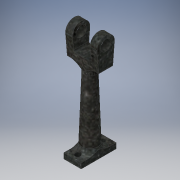
# Autodesk Inventor part: Crankrod
Saved by Autodesk Inventor 2017 (Build 210142000, 142)
## iProperties
Created: 2018-11-07
Part Number: Crankrod
Material: Steel
Document SubType Name: Modeling
Designer: 623516
Density: 7.85 g/cm^3
Appearance: Plate
Author: 623516
Autodesk Inventor part; units mm, degrees
ref_plane "YZ Plane" through (0, 0, 0) normal (1, 0, 0) x (0, 1, 0)
sketch "Sketch1" plane through (0, 0, 0) normal (0, 1, 0) x (-1, 0, 0)
  line L0 (0, 0) -> (10, 0)
  line L1 (10, 0) -> (10, 20)
  line L2 (10, 20) -> (0, 20)
  line L3 (0, 20) -> (0, 0)
  dimension "d0" = 10
  dimension "d1" = 20
  constraints: 8 end point, 2 parallel, 1 horizontal, 1 perpendicular
  measures "d0" distance of L2.end L1.end
  measures "d1" distance of L1.end L0.end
extrude "Extrusion1" add sketch "Sketch1" along normal blind 3
sketch "Sketch2" plane through (0, 3, 0) normal (0, 1, 0) x (1, 0, 0)
  line L0 (-10, 0) -> (-10, -20) construction
  line L1 (-10, -10) -> (0, -10) construction
  line L2 (0, -20) -> (0, 0) construction
  line L3 (-5, -10) -> (-5, -3) construction
  line L4 (-5, -10) -> (-5, -17) construction
  circle A0 centre (-5, -17) radius 1.5 construction
  circle A1 centre (-5, -3) radius 1.5 construction
  circle A2 centre (-5, -17) radius 1.5
  circle A3 centre (-5, -3) radius 1.5
  dimension "d4" = 7
  dimension "d5" = 7
  dimension "d6" = 3
  dimension "d7" = 3
  constraints: 6 end point, 4 centre point, 4 coincident, 3 midpoint, 2 equal radius, 2 vertical
  measures "d4" distance of L3.start L3.end
  measures "d5" distance of L3.start L4.end
  measures "d6" diameter of A0
  measures "d7" diameter of A1
extrude "Extrusion2" cut sketch "Sketch2" against normal blind 3
sketch "Sketch3" plane through (0, 3, 0) normal (0, 1, 0) x (1, 0, 0)
  line L0 (-10, 0) -> (-10, -20) construction
  line L1 (-10, -10) -> (0, -10) construction
  line L2 (0, -20) -> (0, 0) construction
  line L3 (0, 0) -> (-10, 0) construction
  line L4 (-5, 0) -> (-5, -20) construction
  line L5 (-10, -20) -> (0, -20) construction
  circle A0 centre (-5, -10) radius 4.75 construction
  circle A1 centre (-5, -10) radius 4.75
  dimension "d10" = 9.5
  constraints: 5 midpoint, 4 end point, 2 centre point, 1 coincident, 1 concentric
  measures "d10" diameter of A0
ref_plane "Work Plane1" through (0, 46, 0) normal (0, 1, 0) x (1, 0, 0)
sketch "Sketch4" plane through (0, 46, 0) normal (0, 1, 0) x (1, 0, 0)
  line L0 (-10, 0) -> (-10, -20) construction
  line L1 (-10, -10) -> (0, -10) construction
  line L2 (0, -20) -> (0, 0) construction
  line L3 (-5, 0) -> (-5, -20) construction
  line L4 (-10, -20) -> (0, -20) construction
  circle A0 centre (-5, -10) radius 3.25 construction
  circle A1 centre (-5, -10) radius 3.25
  dimension "d12" = 6.5
  dimension "d13" = 20
  constraints: 4 end point, 4 midpoint, 2 centre point, 1 coincident, 1 concentric, 1 parallel
  measures "d12" diameter of A0
  measures "d13" distance from line of L3.start L4
loft "Loft1" add profiles "Sketch4", "Sketch3"
fillet "Fillet1" radius 3 1 edges at (-9.75, 3, 10)
sketch "Sketch6" plane through (-5, 46, 10) normal (0, 1, 0) x (1, 0, 0)
  line L0 (-9, -4) -> (9, -4) construction
  line L1 (9, -4) -> (9, 4) construction
  line L2 (9, 4) -> (-9, 4) construction
  line L3 (-9, 4) -> (-9, -4) construction
  line L4 (-9, -4) -> (9, 4) construction
  line L5 (9, -4) -> (-9, 4) construction
  line L6 (9, 4) -> (-9, 4)
  line L7 (-9, 4) -> (-9, -4)
  line L8 (-9, -4) -> (9, -4)
  line L9 (9, -4) -> (9, 4)
  line L10 (9, 4) -> (-9, -4) construction
  line L11 (-9, 4) -> (9, -4) construction
  point P0 (5, 10)
  point P1 (0, 0)
  point P2 (0, 0)
  dimension "d21" = 18
  dimension "d22" = 8
  dimension "d23" = 4
  dimension "d24" = 6
  constraints: 24 end point, 5 midpoint, 4 parallel, 2 horizontal, 2 perpendicular
  measures "d21" distance of L2.end L1.end
  measures "d22" distance of L1.end L0.end
  measures "d23" distance from line of point (5, 10) L1
  measures "d24" distance from line of point (5, 10) L2
extrude "Extrusion3" add sketch "Sketch6" along normal blind 4
sketch "Sketch7" plane through (4, 46, 14) normal (1, 0, 0) x (0, 0, -1)
  line L0 (0.75, 0) -> (7.25, 0) projected
  circle A0 centre (4, 12) radius 3
  arc A1 (8.931, 11.1724) -> (-0.931, 11.1724) centre (4, 12) ccw
  line L1 (0, 0) -> (0, 4) projected
  line L2 (-1, 12) -> (0, 0)
  line L3 (8, 0) -> (8, 4) projected
  line L4 (8, 0) -> (9, 12)
  line L5 (8, 4) -> (0, 4) projected
  line L6 (0, 0) -> (8, 0) projected
  line L7 (0, 4) -> (0, 0)
  line L8 (8, 0) -> (8, 4)
  line L9 (0, 4) -> (8, 4)
  line L10 (-0.3333, 4) -> (0, 4)
  line L11 (8, 4) -> (8.3333, 4)
  point P0 (14, -46)
  dimension "d28" = 6
  dimension "d29" = 10
  dimension "d30" = 4.764
  dimension "d31" = 4.764
  dimension "d32" = 1
  dimension "d33" = 4
  constraints: 14 end point, 5 point on line, 4 point on circle, 2 centre point, 1 coincident, 1 collinear, 1 horizontal, 1 perpendicular, 1 vertical
  measures "d28" diameter of A0
  measures "d29" diameter of A1
  measures "d30" angle of L3 L4
  measures "d31" angle of L3 L2
  measures "d32" distance from line of L4.end L3
  measures "d33" distance from line of A0.centre L3
extrude "Extrusion4" add sketch "Sketch7" against normal blind 4 contours L10 L2 A1 L4 L11 L5
extrude "Extrusion5" add sketch "Sketch7" against normal blind 9 contours L2 L10 L1 | L3 L11 L4
ref_plane "Work Plane2" through (-5, 46, 14) normal (-1, 0, 0) x (0, 0, 1)
mirror "Mirror1" about plane through (-5, 46, 14) normal (-1, 0, 0) of "Extrusion5", "Extrusion4"
fillet "Fillet2" radius 5 1 edges at (-8.25, 46, 10)
fillet "Fillet3" radius 1 2 edges at (-10, 50, 10) (0, 50, 10)
body "Solid1"
